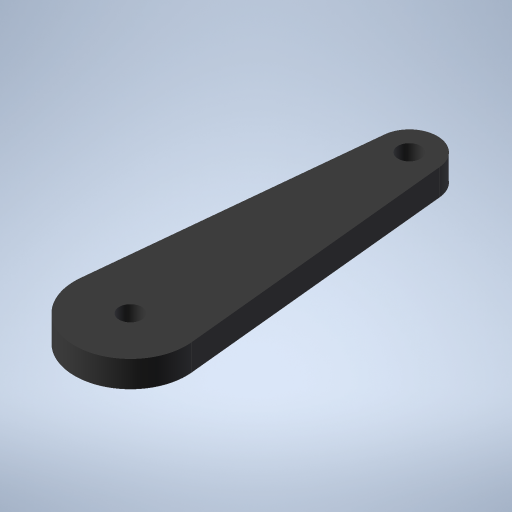
# Autodesk Inventor part: spacing test
Saved by Autodesk Inventor 2024 (Build 280153000, 153)
## iProperties
Created: 2024-04-02
Part Number: spacing test
Material: Generic
Document SubType Name: Modeling
Designer: drew
Density: 1 g/cm^3
Appearance: Default
Author: drew
Autodesk Inventor part; units mm, degrees
ref_plane "YZ Plane" through (0, 0, 0) normal (1, 0, 0) x (0, 1, 0)
ref_plane "XZ Plane" through (0, 0, 0) normal (0, 1, 0) x (-1, 0, 0)
ref_plane "XY Plane" through (0, 0, 0) normal (0, 0, 1) x (1, 0, 0)
sketch "Sketch1" plane through (0, 0, 0) normal (0, 1, 0) x (-1, 0, 0)
  arc A0 (12.6692, -1.2729) -> (-12.6692, -1.2729) centre (0, 0) ccw
  circle A1 centre (0, 0) radius 2.6
  arc A2 (-6.3346, -64.3194) -> (6.3346, -64.3194) centre (0, -63.6829) ccw
  circle A3 centre (0, -63.6829) radius 2.6
  line L0 (12.6692, -1.2729) -> (6.3346, -64.3194)
  line L1 (-12.6692, -1.2729) -> (-6.3346, -64.3194)
  dimension "d0" = 25.466
  dimension "d5" = 5.2
  dimension "d6" = 12.733
  dimension "d8" = 5.2
  dimension "d10" = 63.6829
  constraints: 4 centre point, 4 end point, 4 point on circle, 4 tangent, 3 coincident, 1 vertical alignment
  measures "d0" diameter of A0
  measures "d5" diameter of A1
  measures "d6" diameter of A2
  measures "d8" diameter of A3
  measures "d10" distance of A1.centre A3.centre
extrude "Extrusion1" add sketch "Sketch1" along normal blind 6
body "Solid1"
